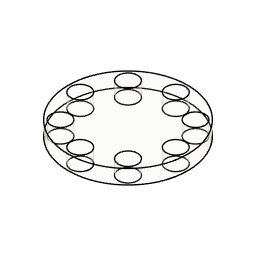
[J,L]C-578VA Joint Spacer (Autodesk Fusion 360 design; units mm, degrees)
Autodesk Fusion 360 part; units mm, degrees
sketch "スケッチ1" plane through (0, 0, 0) normal (0, 0, 1) x (1, 0, 0)
  circle A0 centre (0, 0) radius 12.5
  circle A1 centre (7.0711, 7.0711) radius 2
  circle A2 centre (0, 10) radius 2
  circle A3 centre (-7.0711, 7.0711) radius 2
  circle A4 centre (10, 0) radius 2
  circle A5 centre (-10, 0) radius 2
  circle A6 centre (7.0711, -7.0711) radius 2
  circle A7 centre (0, -10) radius 2
  circle A8 centre (-7.0711, -7.0711) radius 2
  dimension "d2" = 4
  dimension "d3" = 4
  dimension "d4" = 4
  dimension "d5" = 4
  dimension "d6" = 4
  dimension "d7" = 4
  dimension "d8" = 4
  dimension "d9" = 4
  measures "d2" diameter of A1
  measures "d3" diameter of A2
  measures "d4" diameter of A3
  measures "d5" diameter of A4
  measures "d6" diameter of A5
  measures "d7" diameter of A6
  measures "d8" diameter of A7
  measures "d9" diameter of A8
extrude "押し出し1" add sketch "スケッチ1" along normal blind 3
